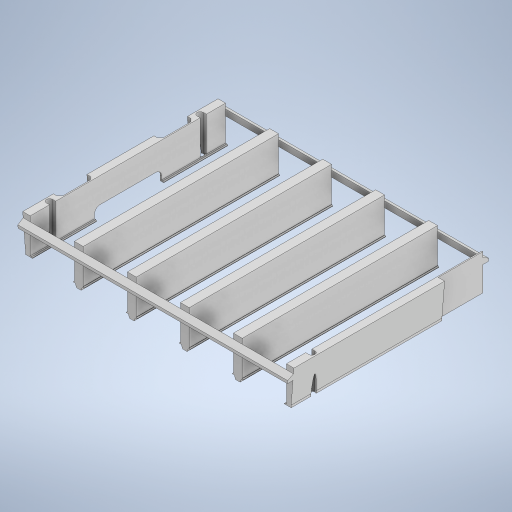
# Autodesk Inventor part: Brackets
Saved by Autodesk Inventor 2023 (Build 270158000, 158)
## iProperties
Created: 2024-03-26
Part Number: Brackets
Material: Generic
Document SubType Name: Modeling
Designer: noname
Density: 1 g/cm^3
Appearance: Default
Author: noname
Autodesk Inventor part; units mm, degrees
ref_plane "YZ Plane" through (0, 0, 0) normal (1, 0, 0) x (0, 1, 0)
ref_plane "XZ Plane" through (0, 0, 0) normal (0, 1, 0) x (-1, 0, 0)
ref_plane "XY Plane" through (0, 0, 0) normal (0, 0, 1) x (1, 0, 0)
sketch "Sketch1" plane through (0, 0, 0) normal (0, 1, 0) x (-1, 0, 0)
  line L0 (0, 0) -> (-97.2, 0) construction
  line L1 (-97.2, 0) -> (-97.2, -70) construction
  line L2 (-97.2, -70) -> (0, -70) construction
  line L3 (0, -70) -> (0, 0) construction
  line L4 (0, 0) -> (-2.7, 0)
  line L5 (-2.7, 0) -> (-2.7, -70)
  line L6 (-2.7, -70) -> (0, -70)
  line L7 (0, -70) -> (0, 0)
  line L8 (-48.6, 0) -> (-48.6, -70)
  line L9 (-97.2, -70) -> (-97.2, 0) construction
  line L10 (-97.2, 0) -> (-94.5, 0)
  line L11 (-94.5, 0) -> (-94.5, -70)
  line L12 (-94.5, -70) -> (-97.2, -70)
  line L13 (-97.2, -70) -> (-97.2, 0)
  line L14 (-18.5, 0) -> (-21.7, 0)
  line L15 (-21.7, 0) -> (-21.7, -70)
  line L16 (-21.7, -70) -> (-18.5, -70)
  line L17 (-18.5, -70) -> (-18.5, 0)
  line L18 (-40.7, 0) -> (-40.7, -70)
  line L19 (-40.7, -70) -> (-37.5, -70)
  line L20 (-37.5, -70) -> (-37.5, 0)
  line L21 (-37.5, 0) -> (-40.7, 0)
  line L22 (-59.7, 0) -> (-59.7, -70)
  line L23 (-59.7, -70) -> (-56.5, -70)
  line L24 (-56.5, -70) -> (-56.5, 0)
  line L25 (-56.5, 0) -> (-59.7, 0)
  line L26 (-78.7, 0) -> (-78.7, -70)
  line L27 (-78.7, -70) -> (-75.5, -70)
  line L28 (-75.5, -70) -> (-75.5, 0)
  line L29 (-75.5, 0) -> (-78.7, 0)
  dimension "d0" = 97.2
  dimension "d1" = 70
  dimension "d2" = 2.7
  dimension "d5" = 19
  dimension "d10" = 19
  dimension "d11" = 3.2
  dimension "d12" = 19
  constraints: 60 end point, 6 parallel, 4 horizontal, 4 symmetric about line, 3 perpendicular, 3 point on line, 2 midpoint, 24 other
  measures "d0" distance between parallel lines of L1 L3
  measures "d1" distance between parallel lines of L0 L2
  measures "d2" distance between parallel lines of L7 L5
  measures "d5" distance of L15.end L18.end
  measures "d10" distance between parallel lines of L5 L15
  measures "d11" distance between parallel lines of L15 L17
  measures "d12" distance between parallel lines of L28 L11
extrude "Extrusion1" add sketch "Sketch1" along normal blind 12
sketch "Sketch2" plane through (0, 0, 0) normal (0, 0, 1) x (1, 0, 0)
  line L0 (18.5, 0) -> (21.7, 0) projected
  line L1 (21.7, 0) -> (21.7, 12) projected
  line L2 (18.5, 12) -> (21.7, 12) projected
  line L3 (18.5, 0) -> (18.5, 12) projected
  line L4 (21.7, 0) -> (18.5, 0) projected
  line L5 (18.5, 0) -> (19.3, -2)
  line L6 (19.3, -2) -> (20.9, -2)
  line L7 (20.9, -2) -> (21.7, 0)
  line L8 (18.5, 0) -> (21.7, 0)
  line L9 (37.5, 0) -> (38.3, -2)
  line L10 (38.3, -2) -> (39.9, -2)
  line L11 (39.9, -2) -> (40.7, 0)
  line L12 (37.5, 0) -> (40.7, 0)
  line L13 (56.5, 0) -> (57.3, -2)
  line L14 (57.3, -2) -> (58.9, -2)
  line L15 (58.9, -2) -> (59.7, 0)
  line L16 (56.5, 0) -> (59.7, 0)
  line L17 (75.5, 0) -> (76.3, -2)
  line L18 (76.3, -2) -> (77.9, -2)
  line L19 (77.9, -2) -> (78.7, 0)
  line L20 (75.5, 0) -> (78.7, 0)
  dimension "d17" = 2
  dimension "d18" = 1.6
  dimension "d21" = 19
  constraints: 32 end point, 2 horizontal, 1 equal length, 1 parallel, 24 other
  measures "d17" distance between parallel lines of L0 L6
  measures "d18" distance of L5.end L6.end
  measures "d21" distance of L0.start L9.start
extrude "Extrusion2" add sketch "Sketch2" against normal up to surface (70 mm away) contours L0 L7 L6 L5 | L12 L11 L10 L9 | L16 L15 L14 L13 | L20 L19 L18 L17
sketch "Sketch3" plane through (0, 0, 0) normal (0, 0, 1) x (1, 0, 0)
  line L0 (0, 12) -> (1, 0)
  line L1 (0, 0) -> (0, 12) projected
  line L2 (0, 12) -> (0, 0)
  line L3 (0, 0) -> (1, 0)
  line L4 (40.7, 0) -> (40.7, 12) projected
  line L5 (40.7, 6) -> (56.5, 6) construction
  line L6 (56.5, 0) -> (56.5, 12) projected
  line L7 (48.6, 12) -> (48.6, 0)
  line L8 (97.2, 12) -> (96.2, 0)
  line L9 (97.2, 0) -> (97.2, 12)
  line L10 (97.2, 0) -> (96.2, 0)
  point P0 (48.6, 6)
  dimension "d28" = 1
  constraints: 16 end point, 4 midpoint, 3 symmetric about line, 2 horizontal alignment, 2 vertical, 1 perpendicular
  measures "d28" distance from line of L1 L0.end
extrude "Extrusion3" cut sketch "Sketch3" against normal through all
ref_plane "Work Plane1" through (0, 9, 0) normal (0, 1, 0) x (1, 0, 0)
sketch "Sketch4" plane through (0, 9, 0) normal (0, 1, 0) x (1, 0, 0)
  line L0 (0, 0) -> (2.7, 0) projected
  line L1 (0, 0) -> (97.2, 0)
  line L2 (97.2, 0) -> (97.2, -2)
  line L3 (97.2, -2) -> (0, -2)
  line L4 (0, -2) -> (0, 0)
  line L5 (2.7, 70) -> (0, 70) projected
  line L6 (0, 70) -> (97.2, 70)
  line L7 (97.2, 70) -> (97.2, 72)
  line L8 (97.2, 72) -> (0, 72)
  line L9 (0, 72) -> (0, 70)
  dimension "d32" = 2
  dimension "d36" = 2
  constraints: 16 end point, 4 parallel, 2 horizontal, 2 perpendicular, 2 vertical alignment
  measures "d32" distance between parallel lines of L6 L8
  measures "d36" distance between parallel lines of L3 L1
extrude "Extrusion4" add sketch "Sketch4" against normal blind 1
draft "FaceDraft1" angle 30 pull direction (0, 0, -1) faces at (38.5667, 9, -71.3333) fixed edges at (48.6, 9, -72)
draft "FaceDraft2" angle 30 pull direction (0, 0, 1) faces at (51.2333, 9, 1.3333) fixed edges at (48.6, 9, 2)
sketch "Sketch5" plane through (1, 0, 0) normal (0, 0, 1) x (1, 0, 0)
  line L0 (-0.6667, 8) -> (-0.8462, 10.1547) projected
  line L1 (-1, 10.1547) -> (-0.8462, 10.1547) projected
  line L2 (-1, 10.1547) -> (-1, 8) projected
  line L3 (-0.6667, 8) -> (-1, 8) projected
  line L4 (96.0462, 10.1547) -> (95.8667, 8) projected
  line L5 (96.2, 8) -> (95.8667, 8) projected
  line L6 (96.2, 10.1547) -> (96.2, 8) projected
  line L7 (96.0462, 10.1547) -> (96.2, 10.1547) projected
  point P0 (-1, 0)
extrude "Extrusion5" cut sketch "Sketch5" along normal through all both and the other way through all
sketch "Sketch6" plane through (0, 12, 0) normal (0, 1, 0) x (1, 0, 0)
  line L0 (97.2, 0) -> (97.2, 70) projected
  line L1 (0.3333, 72) -> (96.8667, 72) projected
  line L2 (97.2, 54) -> (94.9, 54)
  line L3 (94.9, 54) -> (94.9, 72)
  line L4 (94.9, 72) -> (97.2, 72)
  line L5 (97.2, 72) -> (97.2, 54)
  line L6 (94.5, 70) -> (94.5, 0) projected
  point P0 (0, 0)
  dimension "d40" = 0.4
  dimension "d41" = 18
  constraints: 8 end point, 2 parallel, 2 point on line, 1 horizontal, 1 perpendicular
  measures "d40" distance between parallel lines of L6 L3
  measures "d41" distance between parallel lines of L1 L2
extrude "Extrusion6" cut sketch "Sketch6" against normal through all
sketch "Sketch7" plane through (0, 12, 0) normal (0, 1, 0) x (1, 0, 0)
  line L0 (0, 70) -> (0, 0) projected
  line L1 (0, 11) -> (2.3, 11)
  line L2 (2.3, 11) -> (2.3, 23)
  line L3 (2.3, 23) -> (0, 23)
  line L4 (0, 23) -> (0, 11)
  line L5 (0, 47) -> (2.3, 47)
  line L6 (2.3, 47) -> (2.3, 59)
  line L7 (2.3, 59) -> (0, 59)
  line L8 (0, 59) -> (0, 47)
  line L9 (2.7, 70) -> (0, 70) projected
  line L10 (0, 0) -> (2.7, 0) projected
  line L11 (2.7, 0) -> (2.7, 70) projected
  point P0 (1.35, 70)
  point P1 (0, 59)
  point P2 (0, 23)
  dimension "d45" = 11
  dimension "d47" = 11
  dimension "d50" = 0.4
  dimension "d63" = 12
  dimension "d64" = 12
  constraints: 16 end point, 4 parallel, 2 horizontal, 2 perpendicular, 2 point on line, 1 midpoint, 1 vertical alignment
  measures "d45" distance between parallel lines of L7 L9
  measures "d47" distance between parallel lines of L1 L10
  measures "d50" distance between parallel lines of L11 L6
  measures "d63" distance between parallel lines of L5 L7
  measures "d64" distance between parallel lines of L3 L1
extrude "Extrusion7" cut sketch "Sketch7" against normal through all contours L7 L6 L5 L0 | L3 L2 L1 L0
sketch "Sketch8" plane through (0, 0, 0) normal (0, -1, 0) x (1, 0, 0)
  line L0 (2.7, 0) -> (2.7, -70) projected
  line L1 (0, -47) -> (0, -23) projected
  line L2 (2.7, -47.5) -> (0, -47.5)
  line L3 (0, -47.5) -> (0, -22.5)
  line L4 (0, -22.5) -> (2.7, -22.5)
  line L5 (2.7, -22.5) -> (2.7, -47.5)
  line L6 (2.3, -23) -> (1, -23) projected
  line L7 (0, -23) -> (2.3, -23) projected
  line L8 (1, -23) -> (0, -23) projected
  line L9 (0, -47) -> (1, -47) projected
  line L10 (1, -47) -> (2.3, -47) projected
  line L11 (0, -47) -> (1, -47) projected
  line L12 (2.3, -47) -> (0, -47) projected
  line L13 (2.3, -47) -> (2.3, -59) projected
  line L14 (2.3, -59) -> (2.3, -47) projected
  line L15 (2.3, -11) -> (2.3, -23) projected
  line L16 (2.3, -23) -> (2.3, -11) projected
  line L17 (2.3, -23) -> (2.7, -23)
  line L18 (2.3, -47) -> (2.7, -47)
  point P0 (0, 0)
  point P1 (2.7, -35)
  point P2 (2.7, -22.5)
  point P3 (0, -47.5)
  point P4 (0, -23)
  point P5 (0, -47)
  point P6 (2.7, -47)
  point P7 (2.7, -23)
  point P8 (1, -23)
  point P9 (0, -23)
  point P10 (1, -47)
  dimension "d53" = 25
  constraints: 12 end point, 5 point on line, 2 midpoint, 2 parallel, 2 perpendicular, 1 horizontal
  measures "d53" distance between parallel lines of L4 L2
extrude "Extrusion8" cut sketch "Sketch8" against normal blind 3 contours L0 L18 L10 L9 L1 L7 L6 L17
fillet "Fillet1" radius 2 2 edges at (2.5, 3, -23) (2.5, 3, -47)
chamfer "Chamfer1" distance 1 angle 45 4 edges at (2.3, 7.5, -47) (2.3, 6, -11) (2.3, 6, -59) (2.3, 7.5, -23)
ref_plane "Work Plane2" through (10.6, 12, -70) normal (-1, 0, 0) x (0, 0, 1)
pattern_of_nothing "Rectangular Pattern1"
ref_plane "Work Plane7" through (58.9, -2, -35) normal (0, 0, -1) x (-1, 0, 0)
sketch "Sketch13" plane through (0, 12, 0) normal (0, 1, 0) x (1, 0, 0)
  line L0 (40.7, 70) -> (56.5, 70) projected
  line L1 (48.6, 70) -> (48.6, 0)
  line L2 (40.7, 0) -> (56.5, 0) projected
  line L3 (0.25, -2) -> (96.95, -2) projected
  line L4 (94.5, 70) -> (94.5, 0) projected
  line L5 (94.5, 35) -> (2.7, 35)
  line L6 (2.7, 25) -> (2.7, 45) projected
  point P0 (0, 0)
  point P1 (95.6, 8)
  point P2 (1.6, 8)
  point P3 (1.6, 62)
  point P4 (97.35, -2)
  dimension "d91" = 94
  dimension "d92" = 54
  constraints: 4 end point, 4 midpoint, 2 symmetric about line, 1 horizontal alignment, 1 vertical alignment
  measures "d91" distance of point (1.6, 8) point (95.6, 8)
  measures "d92" distance of point (1.6, 62) point (1.6, 8)
hole "Hole2" at (95.6, 12, -8) at (1.6, 12, -8) at (1.6, 12, -62) direction (0, -1, 0) diameter 2.2 end through all
sketch "Sketch14" plane through (0, 12, 0) normal (0, 1, 0) x (1, 0, 0)
  circle A0 centre (95.6, 8) radius 1.1 projected
  line L0 (95.6, 6.9) -> (94.5, 6.9)
  line L1 (94.5, 6.9) -> (94.5, 9.1)
  line L2 (94.5, 9.1) -> (95.6, 9.1)
  line L3 (95.6, 9.1) -> (95.6, 6.9)
  arc A1 (2.7, 8) -> (1, 8.922) centre (1.6, 8) ccw projected
  line L4 (1.6, 9.1) -> (2.7, 9.1)
  line L5 (2.7, 9.1) -> (2.7, 6.9)
  line L6 (2.7, 6.9) -> (1.6, 6.9)
  line L7 (1.6, 6.9) -> (1.6, 9.1)
  circle A2 centre (1.6, 62) radius 1.1 projected
  line L8 (2.7, 62) -> (2.7, 70) projected
  line L9 (1.6, 60.9) -> (2.7, 60.9)
  line L10 (2.7, 60.9) -> (2.7, 63.1)
  line L11 (2.7, 63.1) -> (1.6, 63.1)
  line L12 (1.6, 63.1) -> (1.6, 60.9)
  circle A3 centre (1.6, 8) radius 1.1 projected
  line L13 (2.7, 8) -> (2.7, 62) projected
  line L14 (94.5, 8) -> (94.5, 0) projected
  point P0 (0, 0)
  constraints: 24 end point, 6 parallel, 6 point on line, 5 point on circle, 3 horizontal, 3 perpendicular, 1 tangent
extrude "Extrusion11" cut sketch "Sketch14" against normal through all contours L3 A0 | A0 L1 L2 | L0 L1 A0 | A3 L7 A1 | A1 L4 L5 | L5 L6 A3 | A2 L12 | L10 L9 A2 | A2 L11 L8 picked at (95.5184, 7.6425) picked at (1.6816, 8.3575) picked at (2.1969, 61.7006)
sketch "Sketch15" plane through (0, 0, 0) normal (0, -1, 0) x (1, 0, 0)
  line L0 (95.6, -9.1) -> (94.5, -9.1) projected
  line L1 (94.5, -70) -> (94.5, -9.1) projected
  line L2 (94.9, -70) -> (94.5, -70) projected
  line L3 (94.9, -70) -> (94.9, -54) projected
  line L4 (94.9, -54) -> (96.2, -54) projected
  line L5 (96.2, -54) -> (96.2, -8.922) projected
  arc A0 (95.6, -9.1) -> (96.2, -8.922) centre (95.6, -8) ccw projected
  line L6 (94.5, -6.9) -> (95.6, -6.9) projected
  arc A1 (96.2, -7.078) -> (95.6, -6.9) centre (95.6, -8) ccw projected
  line L7 (96.2, -7.078) -> (96.2, 0) projected
  line L8 (94.5, 0) -> (96.2, 0) projected
  line L9 (94.5, -6.9) -> (94.5, 0) projected
  line L10 (1.6, -6.9) -> (2.7, -6.9) projected
  line L11 (2.7, 0) -> (2.7, -6.9) projected
  line L12 (1, 0) -> (2.7, 0) projected
  line L13 (1, 0) -> (1, -7.078) projected
  arc A2 (1.6, -6.9) -> (1, -7.078) centre (1.6, -8) ccw projected
  line L14 (2.7, -63.1) -> (1.6, -63.1) projected
  arc A3 (1, -62.922) -> (1.6, -63.1) centre (1.6, -62) ccw projected
  line L15 (1, -62.922) -> (1, -70) projected
  line L16 (2.7, -70) -> (1, -70) projected
  line L17 (2.7, -63.1) -> (2.7, -70) projected
  line L18 (1.6, -60.9) -> (2.7, -60.9) projected
  line L19 (2.7, -47) -> (2.7, -60.9) projected
  line L20 (2.7, -47) -> (2.3, -47) projected
  line L21 (2.3, -47) -> (2.3, -58) projected
  line L22 (1.3, -59) -> (2.3, -58) projected
  line L23 (1.3, -59) -> (1, -59) projected
  line L24 (1, -59) -> (1, -61.078) projected
  arc A4 (1.6, -60.9) -> (1, -61.078) centre (1.6, -62) ccw projected
  line L25 (2.7, -9.1) -> (1.6, -9.1) projected
  arc A5 (1, -8.922) -> (1.6, -9.1) centre (1.6, -8) ccw projected
  line L26 (1, -8.922) -> (1, -11) projected
  line L27 (1, -11) -> (1.3, -11) projected
  line L28 (2.3, -12) -> (1.3, -11) projected
  line L29 (2.3, -12) -> (2.3, -23) projected
  line L30 (2.3, -23) -> (2.7, -23) projected
  line L31 (2.7, -9.1) -> (2.7, -23) projected
  point P0 (0, 0)
extrude "Extrusion12" add sketch "Sketch15" along normal blind 0.8
sketch "Sketch16" plane through (0, -0.8, 0) normal (0, -1, 0) x (1, 0, 0)
  arc A0 (95.6, -9.1) -> (96.2, -8.922) centre (95.6, -8) ccw projected
  arc A1 (1, -8.922) -> (1.6, -9.1) centre (1.6, -8) ccw projected
  arc A2 (1, -62.922) -> (1.6, -63.1) centre (1.6, -62) ccw projected
  arc A3 (1.6, -63.1) -> (1.6, -60.9) centre (1.6, -62) ccw
  arc A4 (1.6, -9.1) -> (1.6, -6.9) centre (1.6, -8) ccw
  arc A5 (95.6, -6.9) -> (95.6, -9.1) centre (95.6, -8) ccw
  line L0 (95.6, -9.1) -> (94.5, -9.1) projected
  line L1 (94.5, -6.9) -> (95.6, -6.9) projected
  line L2 (1.6, -6.9) -> (2.7, -6.9) projected
  line L3 (2.7, -9.1) -> (1.6, -9.1) projected
  line L4 (1.6, -60.9) -> (2.7, -60.9) projected
  line L5 (2.7, -63.1) -> (1.6, -63.1) projected
  line L6 (37.5, -70) -> (21.7, -70) projected
  line L7 (22.1, -70) -> (18.1, -70)
  line L8 (18.1, -70) -> (18.1, 0)
  line L9 (18.1, 0) -> (22.1, 0)
  line L10 (22.1, 0) -> (22.1, -70)
  line L11 (21.7, 0) -> (37.5, 0) projected
  line L12 (37.1, 0) -> (41.1, 0)
  line L13 (41.1, 0) -> (41.1, -70)
  line L14 (41.1, -70) -> (37.1, -70)
  line L15 (37.1, -70) -> (37.1, 0)
  line L16 (56.1, -70) -> (60.1, -70)
  line L17 (60.1, -70) -> (60.1, 0)
  line L18 (60.1, 0) -> (56.1, 0)
  line L19 (56.1, 0) -> (56.1, -70)
  line L20 (75.1, 0) -> (79.1, 0)
  line L21 (79.1, 0) -> (79.1, -70)
  line L22 (79.1, -70) -> (75.1, -70)
  line L23 (75.1, -70) -> (75.1, 0)
  line L24 (76.3, -70) -> (77.9, -70) projected
  line L25 (57.3, -70) -> (58.9, -70) projected
  line L26 (38.3, -70) -> (39.9, -70) projected
  line L27 (19.3, -70) -> (20.9, -70) projected
  line L28 (94.5, -70) -> (93.7, -70)
  line L29 (93.7, -70) -> (93.7, 0)
  line L30 (93.7, 0) -> (94.5, 0)
  line L31 (94.5, 0) -> (94.5, -70)
  line L32 (78.7, 0) -> (94.5, 0) projected
  line L33 (2.7, -70) -> (3.5, -70)
  line L34 (3.5, -70) -> (3.5, 0)
  line L35 (3.5, 0) -> (2.7, 0)
  line L36 (2.7, 0) -> (2.7, -70)
  line L37 (2.7, 0) -> (18.5, 0) projected
  line L38 (18.5, -70) -> (2.7, -70) projected
  line L39 (2.7, -23) -> (2.3, -23) projected
  line L40 (2.7, -23) -> (3.5, -23)
  line L41 (2.3, -47) -> (2.7, -47) projected
  line L42 (2.7, -47) -> (3.5, -47)
  point P0 (0, 0)
  point P1 (77.1, -70)
  point P2 (58.1, -70)
  point P3 (39.1, -70)
  point P4 (20.1, -70)
  dimension "d98" = 4
  dimension "d99" = 0.8
  constraints: 52 end point, 13 point on line, 12 parallel, 8 midpoint, 7 perpendicular, 6 horizontal, 6 point on circle, 4 equal length, 3 centre point, 3 coincident, 1 collinear
  measures "d98" distance between parallel lines of L23 L21
  measures "d99" distance between parallel lines of L31 L29
extrude "Extrusion13" add sketch "Sketch16" against normal blind 0.4 contours A3 L36 L5 | A3 L4 L36 | L36 L42 L34 L33 | L36 L35 L34 L40 | L8 L9 L10 L6 L7 | L3 A4 L36 | A4 L2 L36 | L11 L12 L13 L14 L6 L15 | A5 L31 L1 | L31 L28 L29 L30 | A5 L0 L31 | L19 L18 L17 L16 | L20 L21 L22 L23
sketch "Sketch17" plane through (0, -0.4, 0) normal (0, 1, 0) x (1, 0, 0)
  line L0 (21.7, 0) -> (21.7, 70) projected
  line L1 (21.7, 70) -> (18.5, 70) projected
  line L2 (18.5, 70) -> (18.5, 0) projected
  line L3 (18.5, 0) -> (21.7, 0) projected
  line L4 (40.7, 70) -> (37.5, 70) projected
  line L5 (37.5, 70) -> (37.5, 0) projected
  line L6 (37.5, 0) -> (40.7, 0) projected
  line L7 (40.7, 0) -> (40.7, 70) projected
  line L8 (59.7, 70) -> (56.5, 70) projected
  line L9 (56.5, 70) -> (56.5, 0) projected
  line L10 (56.5, 0) -> (59.7, 0) projected
  line L11 (59.7, 0) -> (59.7, 70) projected
  line L12 (78.7, 70) -> (75.5, 70) projected
  line L13 (75.5, 70) -> (75.5, 0) projected
  line L14 (75.5, 0) -> (78.7, 0) projected
  line L15 (78.7, 0) -> (78.7, 70) projected
  point P0 (0, 0)
extrude "Extrusion14" add sketch "Sketch17" along normal through all
chamfer "Chamfer2" distance 0.3 angle 45 3 edges at (3.5, -0.4, -11.5) (3.5, -0.4, -58.5) (93.7, -0.4, -35)
chamfer "Chamfer3" distance 0.3 angle 45 8 edges at (22.1, -0.4, -35) (18.1, -0.4, -35) (37.1, -0.4, -35) (41.1, -0.4, -35) (56.1, -0.4, -35) (60.1, -0.4, -35) (75.1, -0.4, -35) (79.1, -0.4, -35)
ref_plane "Work Plane3" through (29.6, 12, -70) normal (-1, 0, 0) x (0, 0, 1)
ref_plane "Work Plane4" through (48.6, 12, -70) normal (-1, 0, 0) x (0, 0, 1)
ref_plane "Work Plane5" through (67.6, 12, -70) normal (-1, 0, 0) x (0, 0, 1)
ref_plane "Work Plane6" through (86.6, 12, -70) normal (-1, 0, 0) x (0, 0, 1)
body "Solid1"
